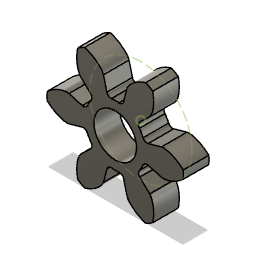
gear (small) middle v2 (Autodesk Fusion 360 design; units mm, degrees)
description: small size, for middle
description: Spur Gear; Module: 2.0; Num Teeth: 6; Pressure Angle: 20.0; Backlash: 0.00 mm
Autodesk Fusion 360 part; units mm, degrees
sketch "草图1" plane through (0, 0, 0) normal (0, 0, 1) x (1, 0, 0) in component "Spur Gear (6 teeth)"
  circle A0 centre (0, 0) radius 3.5492
  circle A1 centre (0, 0) radius 2.5
extrude "拉伸1" add sketch "草图1" along normal blind 3 in component "Spur Gear (6 teeth)"
sketch "草图2" plane through (0, 0, 0) normal (0, 0, 1) x (1, 0, 0) in component "Spur Gear (6 teeth)"
  spline S0 degree 5 poles (5.4237, -1.5403) (5.4306, -1.5422) (5.4444, -1.5458) (5.4654, -1.5503) (5.4937, -1.5547) (5.5295, -1.5577) (5.5656, -1.5592) (5.602, -1.5596) (5.6385, -1.5595) (5.6751, -1.559) (5.7117, -1.558) (5.7485, -1.5565) (5.7854, -1.5541) (5.8224, -1.5509) (5.8596, -1.5469) (5.8968, -1.542) (5.9342, -1.5365) (5.9716, -1.5304) (6.009, -1.5238) (6.0465, -1.5167) (6.084, -1.509) (6.1216, -1.5009) (6.1592, -1.4921) (6.1968, -1.4828) (6.2344, -1.473) (6.2721, -1.4625) (6.3098, -1.4516) (6.3475, -1.4402) (6.3851, -1.4282) (6.4228, -1.4158) (6.4605, -1.403) (6.4982, -1.3896) (6.5358, -1.3757) (6.5734, -1.3614) (6.611, -1.3466) (6.6486, -1.3313) (6.6861, -1.3156) (6.7236, -1.2994) (6.7611, -1.2828) (6.7985, -1.2657) (6.8359, -1.2482) (6.8732, -1.2302) (6.9104, -1.2118) (6.9476, -1.193) (6.9848, -1.1737) (7.0219, -1.154) (7.0589, -1.1339) (7.0958, -1.1133) (7.1326, -1.0923) (7.1694, -1.071) (7.2061, -1.0492) (7.2427, -1.027) (7.2792, -1.0043) (7.3157, -0.9813) (7.352, -0.9579) (7.3882, -0.9341) (7.4244, -0.9098) (7.4604, -0.8852) (7.4963, -0.8602) (7.5321, -0.8348) (7.5678, -0.809) (7.6034, -0.7828) (7.6388, -0.7563) (7.6742, -0.7293) (7.7094, -0.702) (7.7445, -0.6743) (7.7794, -0.6462) (7.8142, -0.6178) (7.8489, -0.589) (7.8834, -0.5598) (7.9178, -0.5303) (7.9452, -0.5063) (7.9657, -0.4882) (7.9794, -0.4761) (7.9862, -0.47) knots 0 0 0 0 0 0 0.01428571 0.02857143 0.04285714 0.05714286 0.07142857 0.08571429 0.1 0.11428571 0.12857143 0.14285714 0.15714286 0.17142857 0.18571429 0.2 0.21428571 0.22857143 0.24285714 0.25714286 0.27142857 0.28571429 0.3 0.31428571 0.32857143 0.34285714 0.35714286 0.37142857 0.38571429 0.4 0.41428571 0.42857143 0.44285714 0.45714286 0.47142857 0.48571429 0.5 0.51428571 0.52857143 0.54285714 0.55714286 0.57142857 0.58571429 0.6 0.61428571 0.62857143 0.64285714 0.65714286 0.67142857 0.68571429 0.7 0.71428571 0.72857143 0.74285714 0.75714286 0.77142857 0.78571429 0.8 0.81428571 0.82857143 0.84285714 0.85714286 0.87142857 0.88571429 0.9 0.91428571 0.92857143 0.94285714 0.95714286 0.97142857 0.98571429 1 1 1 1 1 1
  spline S1 degree 5 poles (5.4237, 1.5403) (5.4306, 1.5422) (5.4444, 1.5458) (5.4654, 1.5503) (5.4937, 1.5547) (5.5295, 1.5577) (5.5656, 1.5592) (5.602, 1.5596) (5.6385, 1.5595) (5.6751, 1.559) (5.7117, 1.558) (5.7485, 1.5565) (5.7854, 1.5541) (5.8224, 1.5509) (5.8596, 1.5469) (5.8968, 1.542) (5.9342, 1.5365) (5.9716, 1.5304) (6.009, 1.5238) (6.0465, 1.5167) (6.084, 1.509) (6.1216, 1.5009) (6.1592, 1.4921) (6.1968, 1.4828) (6.2344, 1.473) (6.2721, 1.4625) (6.3098, 1.4516) (6.3475, 1.4402) (6.3851, 1.4282) (6.4228, 1.4158) (6.4605, 1.403) (6.4982, 1.3896) (6.5358, 1.3757) (6.5734, 1.3614) (6.611, 1.3466) (6.6486, 1.3313) (6.6861, 1.3156) (6.7236, 1.2994) (6.7611, 1.2828) (6.7985, 1.2657) (6.8359, 1.2482) (6.8732, 1.2302) (6.9104, 1.2118) (6.9476, 1.193) (6.9848, 1.1737) (7.0219, 1.154) (7.0589, 1.1339) (7.0958, 1.1133) (7.1326, 1.0923) (7.1694, 1.071) (7.2061, 1.0492) (7.2427, 1.027) (7.2792, 1.0043) (7.3157, 0.9813) (7.352, 0.9579) (7.3882, 0.9341) (7.4244, 0.9098) (7.4604, 0.8852) (7.4963, 0.8602) (7.5321, 0.8348) (7.5678, 0.809) (7.6034, 0.7828) (7.6388, 0.7563) (7.6742, 0.7293) (7.7094, 0.702) (7.7445, 0.6743) (7.7794, 0.6462) (7.8142, 0.6178) (7.8489, 0.589) (7.8834, 0.5598) (7.9178, 0.5303) (7.9452, 0.5063) (7.9657, 0.4882) (7.9794, 0.4761) (7.9862, 0.47) knots 0 0 0 0 0 0 0.01428571 0.02857143 0.04285714 0.05714286 0.07142857 0.08571429 0.1 0.11428571 0.12857143 0.14285714 0.15714286 0.17142857 0.18571429 0.2 0.21428571 0.22857143 0.24285714 0.25714286 0.27142857 0.28571429 0.3 0.31428571 0.32857143 0.34285714 0.35714286 0.37142857 0.38571429 0.4 0.41428571 0.42857143 0.44285714 0.45714286 0.47142857 0.48571429 0.5 0.51428571 0.52857143 0.54285714 0.55714286 0.57142857 0.58571429 0.6 0.61428571 0.62857143 0.64285714 0.65714286 0.67142857 0.68571429 0.7 0.71428571 0.72857143 0.74285714 0.75714286 0.77142857 0.78571429 0.8 0.81428571 0.82857143 0.84285714 0.85714286 0.87142857 0.88571429 0.9 0.91428571 0.92857143 0.94285714 0.95714286 0.97142857 0.98571429 1 1 1 1 1 1
  arc A0 (7.9862, -0.47) -> (7.9862, 0.47) centre (0, 0) ccw
  line L0 (3.4046, -0.9696) -> (5.4237, -1.5403)
  line L1 (3.4046, 0.9696) -> (5.4237, 1.5403)
  line L2 (3.4046, -0.9696) -> (3.4046, 0.9696)
  point P0 (5.5935, -1.5594)
  point P1 (5.7697, -1.555)
  point P2 (5.9497, -1.5339)
  point P3 (6.1326, -1.4982)
  point P4 (6.3176, -1.4491)
  point P5 (6.5041, -1.3873)
  point P6 (6.6914, -1.3132)
  point P7 (6.8792, -1.2272)
  point P8 (7.0668, -1.1294)
  point P9 (7.2538, -1.02)
  point P10 (7.4397, -0.8993)
  point P11 (7.6241, -0.7673)
  point P12 (7.8064, -0.6241)
  point P13 (5.5935, 1.5594)
  point P14 (5.7697, 1.555)
  point P15 (5.9497, 1.5339)
  point P16 (6.1326, 1.4982)
  point P17 (6.3176, 1.4491)
  point P18 (6.5041, 1.3873)
  point P19 (6.6914, 1.3132)
  point P20 (6.8792, 1.2272)
  point P21 (7.0668, 1.1294)
  point P22 (7.2538, 1.02)
  point P23 (7.4397, 0.8993)
  point P24 (7.6241, 0.7673)
  point P25 (7.8064, 0.6241)
extrude "拉伸2" add sketch "草图2" along normal blind 3 in component "Spur Gear (6 teeth)"
fillet "圆角1" radius 0.5 2 edges at (3.4135, -0.9721, 1.5) (3.4135, 0.9721, 1.5) in component "Spur Gear (6 teeth)"
pattern_circular "C-阵列1" count 6 over 360 about axis through (0, 0, 0) along (0, 0, 1) of "拉伸2", "圆角1" in component "Spur Gear (6 teeth)"
sketch "草图3" plane through (0, 0, 0) normal (0, 0, 1) x (1, 0, 0) in component "Spur Gear (6 teeth)"
  circle A0 centre (0, 0) radius 6 construction
component "Spur Gear (6 teeth)" placed x (1, 0, 0) y (0, 1, 0) z (0, 0, 1) at (0, 0, 0)
